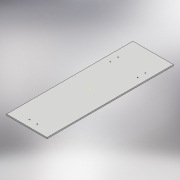
# Autodesk Inventor part: 内层16cm板
Saved by Autodesk Inventor 2017 (Build 210142000, 142)
## iProperties
Part Number: 内层16cm板
Material: 常规
Document SubType Name: 钣金
Designer: PANDA
Density: 1 g/cm^3
Sheet Metal Rule: 默认_mm
Appearance: 默认
Author: PANDA
Autodesk Inventor part; units mm, degrees
ref_plane "YZ Plane" through (0, 0, 0) normal (1, 0, 0) x (0, 1, 0)
ref_plane "XZ Plane" through (0, 0, 0) normal (0, 1, 0) x (-1, 0, 0)
ref_plane "XY Plane" through (0, 0, 0) normal (0, 0, 1) x (1, 0, 0)
sketch "草图16" plane through (0, 0, 0) normal (0, 0, 1) x (1, 0, 0)
  line L0 (-80, 250) -> (80, 250)
  line L1 (80, 250) -> (80, -250)
  line L2 (80, -250) -> (-80, -250)
  line L3 (-80, -250) -> (-80, 250)
  point P0 (0, 0)
  dimension "d46" = 160
  dimension "d47" = 500
  constraints: 8 end point, 2 parallel, 1 horizontal, 1 perpendicular
  measures "d46" distance of L1.end L2.end
  measures "d47" distance of L0.end L1.end
extrude "拉伸16" add sketch "草图16" along normal blind 5
sketch "草图17" plane through (0, 0, 5) normal (0, 0, 1) x (1, 0, 0)
  circle A0 centre (15.5, -224) radius 1.8
  point P0 (0, 0)
  dimension "d50" = 3.6
  constraints: 1 centre point
  measures "d50" diameter of A0
extrude "拉伸17" cut sketch "草图17" against normal through all
sketch "草图18" plane through (0, 0, 5) normal (0, 0, 1) x (1, 0, 0)
  circle A0 centre (-15.5, -224) radius 1.8
  point P0 (0, 0)
  dimension "d53" = 3.6
  constraints: 1 centre point
  measures "d53" diameter of A0
extrude "拉伸18" cut sketch "草图18" against normal through all
sketch "草图23" plane through (0, 0, 5) normal (0, 0, 1) x (1, 0, 0)
  point P0 (0, 0)
sketch "草图24" plane through (0, 0, 5) normal (0, 0, 1) x (1, 0, 0)
  point P0 (0, 0)
sketch "草图25" plane through (0, 0, 5) normal (0, 0, 1) x (1, 0, 0)
  circle A0 centre (54, 165.5) radius 1.8
  point P0 (0, 0)
  dimension "d68" = 3.6
  constraints: 1 centre point
  measures "d68" diameter of A0
extrude "拉伸23" cut sketch "草图25" against normal through all
sketch "草图26" plane through (0, 0, 5) normal (0, 0, 1) x (1, 0, 0)
  circle A0 centre (54, 134.5) radius 1.8
  point P0 (0, 0)
  dimension "d71" = 3.6
  constraints: 1 centre point
  measures "d71" diameter of A0
extrude "拉伸24" cut sketch "草图26" against normal through all
sketch "草图27" plane through (0, 0, 5) normal (0, 0, 1) x (1, 0, 0)
  circle A0 centre (-54, 165.5) radius 1.8
  point P0 (0, 0)
  dimension "d74" = 3.6
  constraints: 1 centre point
  measures "d74" diameter of A0
extrude "拉伸25" cut sketch "草图27" against normal through all
sketch "草图28" plane through (0, 0, 5) normal (0, 0, 1) x (1, 0, 0)
  circle A0 centre (-54, 134.5) radius 1.8
  point P0 (0, 0)
  dimension "d77" = 3.6
  constraints: 1 centre point
  measures "d77" diameter of A0
extrude "拉伸26" cut sketch "草图28" against normal through all
equation "\"折弯半径\" = 厚度"
equation "\"折弯释压宽度\" = 厚度"
equation "\"折弯释压深度\" = 0.5 * 厚度"
equation "\"拐角释压尺寸\" = 4 * 厚度"
equation "\"最小余量\" = 2 * 厚度"
equation "\"过渡半径\" = 折弯半径"
equation "\"Jacobi半径尺寸\" = 折弯半径"
equation "\"间隙大小\" = 厚度"
equation "\"厚度\" = 0.5"
